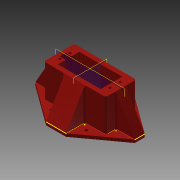
# Autodesk Inventor part: Servo Mount
Saved by Autodesk Inventor 2015 (Build 190159000, 159)
## iProperties
Created: 2016-12-13
Part Number: Servo Mount
Material: Generic
Document SubType Name: Modeling
Designer: Rudge-Top
Density: 1 g/cm^3
Appearance: Orange-Red
Author: Rudge-Top
Autodesk Inventor part; units mm, degrees
ref_plane "YZ Plane" through (0, 0, 0) normal (1, 0, 0) x (0, 1, 0)
ref_plane "XZ Plane" through (0, 0, 0) normal (0, 1, 0) x (-1, 0, 0)
ref_plane "XY Plane" through (0, 0, 0) normal (0, 0, 1) x (1, 0, 0)
sketch "Sketch1" plane through (0, 0, 0) normal (0, 1, 0) x (-1, 0, 0)
  line L0 (0, 0) -> (43, 0)
  line L1 (43, 0) -> (43, -21.5)
  line L2 (43, -21.5) -> (0, -21.5)
  line L3 (0, -21.5) -> (0, 0)
  line L4 (52.5, -26) -> (52.5, 4.5)
  line L5 (-9.5, 4.5) -> (-9.5, -26)
  line L6 (-9.5, 4.5) -> (52.5, 4.5)
  line L7 (52.5, -26) -> (-9.5, -26)
  dimension "d0" = 43
  dimension "d1" = 21.5
  dimension "d2" = 9.5
  dimension "d15" = 4.5
  dimension "d16" = 4.5
  dimension "d49" = 9.5
  constraints: 16 end point, 3 parallel, 3 perpendicular, 1 horizontal
  measures "d0" distance of L1.end L2.end
  measures "d1" distance of L0.end L1.end
  measures "d2" distance between parallel lines of L1 L4
  measures "d15" distance between parallel lines of L2 L7
  measures "d16" distance between parallel lines of L6 L0
  measures "d49" distance between parallel lines of L5 L3
extrude "Extrusion1" add sketch "Sketch1" along normal blind 29.5
sketch "Sketch2" plane through (0, 0, 0) normal (0, -1, 0) x (1, 0, 0)
  line L0 (-52.5, 4.5) -> (9.5, 4.5)
  line L1 (9.5, 4.5) -> (9.5, -26)
  line L2 (9.5, -26) -> (-52.5, -26)
  line L3 (-52.5, -26) -> (-52.5, 4.5)
  point P0 (0, 0)
  constraints: 8 end point, 2 parallel, 1 horizontal, 1 perpendicular
extrude "Extrusion2" add sketch "Sketch2" along normal blind 3
fillet "Fillet1" radius 2 4 edges at (-52.5, 13.25, -26) (9.5, 13.25, -26) (9.5, 13.25, 4.5) (-52.5, 13.25, 4.5)
sketch "Sketch3" plane through (0, 29.5, 0) normal (0, 1, 0) x (1, 0, 0)
  arc A0 (-52.5, -2.5) -> (-50.5, -4.5) centre (-50.5, -2.5) ccw projected
  arc A1 (7.5, -4.5) -> (9.5, -2.5) centre (7.5, -2.5) ccw projected
  line L0 (9.5, -2.5) -> (9.5, 24) projected
  arc A2 (9.5, 24) -> (7.5, 26) centre (7.5, 24) ccw projected
  arc A3 (-50.5, 26) -> (-52.5, 24) centre (-50.5, 24) ccw projected
  line L1 (-52.5, 24) -> (-52.5, -2.5) projected
  line L2 (-43, 0) -> (-43, 21.5) projected
  line L3 (-43, 21.5) -> (0, 21.5) projected
  line L4 (0, 21.5) -> (0, 0) projected
  line L5 (0, 0) -> (-43, 0) projected
  line L6 (-50.5, -4.5) -> (7.5, -4.5) projected
  line L7 (7.5, 26) -> (-50.5, 26) projected
  point P0 (3.5, 5.75)
  point P1 (3.5, 15.75)
  point P2 (-46.5, 5.75)
  point P3 (-46.5, 15.75)
  dimension "d8" = 10
  dimension "d10" = 3.5
  dimension "d11" = 10
  dimension "d12" = 3.5
  dimension "d17" = 10.25
  dimension "d18" = 10.25
  measures "d8" distance of point (-46.5, 5.75) point (-46.5, 15.75)
  measures "d10" distance from line of L2 point (-46.5, 15.75)
  measures "d11" distance of point (3.5, 15.75) point (3.5, 5.75)
  measures "d12" distance from line of L4 point (3.5, 5.75)
  measures "d17" distance from line of L6 point (3.5, 5.75)
  measures "d18" distance from line of L7 point (-46.5, 15.75)
hole "Hole1" at (3.5, 29.5, -5.75) at (3.5, 29.5, -15.75) at (-46.5, 29.5, -5.75) at (-46.5, 29.5, -15.75) direction (0, -1, 0) diameter 2.5 depth 20 tip angle 118
ref_plane "Work Plane1" through (-21.5, -3, 2.5) normal (1, 0, 0) x (0, 0, -1)
sketch "Sketch4" plane through (-21.5, -3, 2.5) normal (1, 0, 0) x (0, 0, -1)
  line L0 (0, 0) -> (0, 32.5) projected
  line L1 (26.5, 0) -> (0, 0) projected
  line L2 (26.5, 32.5) -> (26.5, 0) projected
  line L3 (0, 32.5) -> (26.5, 32.5) projected
  line L4 (28.5, 32.5) -> (26.5, 32.5) projected
  line L5 (26.5, 32.5) -> (26.5, 0) projected
  line L6 (26.5, 0) -> (28.5, 0) projected
  line L7 (28.5, 0) -> (28.5, 32.5) projected
  line L8 (28.5, 32.5) -> (47.2639, 0)
  line L9 (28.5, 32.5) -> (66.0278, 32.5) construction
  line L10 (47.2639, 0) -> (28.5, 0)
  point P0 (2.5, 3)
  dimension "d26" = 60
  constraints: 6 end point, 2 horizontal, 1 equal length
  measures "d26" angle of L8 L9
extrude "Extrusion3" add sketch "Sketch4" along normal mid plane 20 contours L7 L8 L10
ref_plane "Work Plane2" through (-50.5, -3, -10.75) normal (0, 0, -1) x (-1, 0, 0)
mirror "Mirror1" about plane through (-50.5, -3, -10.75) normal (0, 0, -1) of "Extrusion3"
sketch "Sketch5" plane through (-50.5, -3, -10.75) normal (0, 0, -1) x (-1, 0, 0)
  line L0 (-58, 32.5) -> (-60, 32.5) projected
  line L1 (-60, 32.5) -> (-60, 0) projected
  line L2 (-60, 0) -> (-58, 0) projected
  line L3 (-58, 0) -> (-58, 32.5) projected
  line L4 (-60, 32.5) -> (-78.7639, 0)
  line L5 (-60, 32.5) -> (-22.4722, 32.5) construction
  line L6 (-78.7639, 0) -> (-60, 0)
  line L7 (-60, 32.5) -> (-60, 0)
  point P0 (-50.5, 3)
  dimension "d29" = 240
  constraints: 8 end point, 2 horizontal, 1 collinear, 1 equal length
extrude "Extrusion4" add sketch "Sketch5" along normal mid plane 10 contours L1 L6 L4
mirror "Mirror2" about plane through (-21.5, -3, 2.5) normal (1, 0, 0) of "Extrusion4"
fillet "Fillet2" radius 2 8 edges at (9.5, 13.25, -15.75) (9.5, 13.25, -5.75) (-11.5, 13.25, -26) (-31.5, 13.25, -26) (-52.5, 13.25, -15.75) (-52.5, 13.25, -5.75) (-31.5, 13.25, 4.5) (-11.5, 13.25, 4.5)
sketch "Sketch6" plane through (0, -3, 0) normal (0, -1, 0) x (1, 0, 0)
  line L0 (-43, -21.5) -> (0, -21.5)
  line L1 (0, -21.5) -> (0, 0)
  line L2 (0, 0) -> (-43, 0)
  line L3 (-43, 0) -> (-43, -21.5)
  line L4 (-50.5, -26) -> (-33.5, -26) projected
  line L5 (-52.5, 2.5) -> (-52.5, -3.75) projected
  point P0 (0, 0)
  dimension "d33" = 43
  dimension "d34" = 21.5
  dimension "d35" = 4.5
  dimension "d36" = 9.5
  constraints: 8 end point, 2 parallel, 1 horizontal, 1 perpendicular
  measures "d33" distance of L2.end L1.end
  measures "d34" distance of L1.end L0.end
  measures "d35" distance between parallel lines of L4 L0
  measures "d36" distance between parallel lines of L5 L3
extrude "Extrusion5" cut sketch "Sketch6" against normal blind 3
sketch "Sketch7" plane through (0, 29.5, 0) normal (0, 1, 0) x (1, 0, 0)
  circle A0 centre (-46.5, 5.75) radius 1.25 projected
  circle A1 centre (3.5, 5.75) radius 1.25 projected
  circle A2 centre (3.5, 15.75) radius 1.25 projected
  circle A3 centre (-46.5, 15.75) radius 1.25 projected
  arc A4 (-52.5, -2.5) -> (-50.5, -4.5) centre (-50.5, -2.5) ccw projected
  line L0 (-50.5, -4.5) -> (-33.5, -4.5) projected
  line L1 (-33.5, -4.5) -> (-9.5, -4.5) projected
  line L2 (-9.5, -4.5) -> (7.5, -4.5) projected
  arc A5 (7.5, -4.5) -> (9.5, -2.5) centre (7.5, -2.5) ccw projected
  line L3 (9.5, -2.5) -> (9.5, 3.75) projected
  line L4 (9.5, 3.75) -> (9.5, 17.75) projected
  line L5 (9.5, 17.75) -> (9.5, 24) projected
  arc A6 (9.5, 24) -> (7.5, 26) centre (7.5, 24) ccw projected
  line L6 (7.5, 26) -> (-9.5, 26) projected
  line L7 (-9.5, 26) -> (-33.5, 26) projected
  line L8 (-33.5, 26) -> (-50.5, 26) projected
  arc A7 (-50.5, 26) -> (-52.5, 24) centre (-50.5, 24) ccw projected
  line L9 (-52.5, 24) -> (-52.5, 17.75) projected
  line L10 (-52.5, 17.75) -> (-52.5, 3.75) projected
  line L11 (-52.5, 3.75) -> (-52.5, -2.5) projected
  line L12 (-43, 0) -> (-43, 21.5) projected
  line L13 (-43, 21.5) -> (0, 21.5) projected
  line L14 (0, 21.5) -> (0, 0) projected
  line L15 (0, 0) -> (-43, 0) projected
  line L16 (-43, 13.75) -> (-49, 13.75)
  line L17 (-49, 13.75) -> (-49, 7.75)
  line L18 (-49, 7.75) -> (-43, 7.75)
  line L19 (-43, 7.75) -> (-43, 13.75)
  line L20 (-43, 10.75) -> (-46.1833, 10.75)
  line L21 (-43, 10.75) -> (-39.8167, 10.75) construction
  dimension "d39" = 6
  dimension "d40" = 6
  dimension "d41" = 180
  dimension "d51" = 7.75
  dimension "d52" = 7.75
  constraints: 12 end point, 2 horizontal, 2 parallel, 1 collinear, 1 midpoint, 1 perpendicular, 1 point on line
  measures "d39" distance of L18.end L17.end
  measures "d40" distance of L17.end L16.end
  measures "d41" angle of L20 L21
  measures "d51" distance from line of L13 L16.start
  measures "d52" distance from line of L15 L18.end
extrude "Extrusion6" cut sketch "Sketch7" against normal blind 40 contours L18 L17 L16 L12
fillet "Fillet3" radius 0.5 2 edges at (-43, 13.25, -13.75) (-43, 13.25, -7.75)
fillet "Fillet4" radius 0.5 4 edges at (0, 13.25, -21.5) (0, 13.25, 0) (-43, 13.25, -21.5) (-43, 13.25, 0)
sketch "Sketch8" plane through (0, -3, 0) normal (0, -1, 0) x (1, 0, 0)
  arc A0 (-50.5, 4.5) -> (-52.5, 2.5) centre (-50.5, 2.5) ccw projected
  line L0 (-52.5, 2.5) -> (-52.5, -3.75) projected
  arc A1 (-54.5, -5.75) -> (-52.5, -3.75) centre (-54.5, -3.75) ccw projected
  line L1 (-54.5, -5.75) -> (-71.2639, -5.75) projected
  line L2 (-71.2639, -5.75) -> (-71.2639, -15.75) projected
  line L3 (-71.2639, -15.75) -> (-54.5, -15.75) projected
  arc A2 (-52.5, -17.75) -> (-54.5, -15.75) centre (-54.5, -17.75) ccw projected
  line L4 (-52.5, -17.75) -> (-52.5, -24) projected
  arc A3 (-52.5, -24) -> (-50.5, -26) centre (-50.5, -24) ccw projected
  line L5 (-50.5, -26) -> (-33.5, -26) projected
  arc A4 (-31.5, -28) -> (-33.5, -26) centre (-33.5, -28) ccw projected
  line L6 (-31.5, -44.7639) -> (-31.5, -28) projected
  line L7 (-31.5, -44.7639) -> (-11.5, -44.7639) projected
  line L8 (-11.5, -28) -> (-11.5, -44.7639) projected
  arc A5 (-9.5, -26) -> (-11.5, -28) centre (-9.5, -28) ccw projected
  line L9 (-9.5, -26) -> (7.5, -26) projected
  arc A6 (7.5, -26) -> (9.5, -24) centre (7.5, -24) ccw projected
  line L10 (9.5, -24) -> (9.5, -17.75) projected
  arc A7 (11.5, -15.75) -> (9.5, -17.75) centre (11.5, -17.75) ccw projected
  line L11 (28.2639, -15.75) -> (11.5, -15.75) projected
  line L12 (28.2639, -5.75) -> (28.2639, -15.75) projected
  line L13 (11.5, -5.75) -> (28.2639, -5.75) projected
  arc A8 (9.5, -3.75) -> (11.5, -5.75) centre (11.5, -3.75) ccw projected
  line L14 (9.5, -3.75) -> (9.5, 2.5) projected
  arc A9 (9.5, 2.5) -> (7.5, 4.5) centre (7.5, 2.5) ccw projected
  line L15 (7.5, 4.5) -> (-9.5, 4.5) projected
  arc A10 (-11.5, 6.5) -> (-9.5, 4.5) centre (-9.5, 6.5) ccw projected
  line L16 (-11.5, 6.5) -> (-11.5, 23.2639) projected
  line L17 (-31.5, 23.2639) -> (-11.5, 23.2639) projected
  line L18 (-31.5, 23.2639) -> (-31.5, 6.5) projected
  arc A11 (-33.5, 4.5) -> (-31.5, 6.5) centre (-33.5, 6.5) ccw projected
  line L19 (-33.5, 4.5) -> (-50.5, 4.5) projected
  line L20 (-43, -7.25) -> (-43, -0.5) projected
  arc A12 (-42.5, 0) -> (-43, -0.5) centre (-42.5, -0.5) ccw projected
  line L21 (-42.5, 0) -> (-0.5, 0) projected
  arc A13 (0, -0.5) -> (-0.5, 0) centre (-0.5, -0.5) ccw projected
  line L22 (0, -0.5) -> (0, -21) projected
  arc A14 (-0.5, -21.5) -> (0, -21) centre (-0.5, -21) ccw projected
  line L23 (-0.5, -21.5) -> (-42.5, -21.5) projected
  arc A15 (-43, -21) -> (-42.5, -21.5) centre (-42.5, -21) ccw projected
  line L24 (-43.5, -13.75) -> (-49, -13.75) projected
  line L25 (-49, -13.75) -> (-49, -7.75) projected
  line L26 (-49, -7.75) -> (-43.5, -7.75) projected
  line L27 (-49, -13.75) -> (-71.2639, -13.75)
  line L28 (-71.2639, -13.75) -> (-71.2639, -7.75)
  line L29 (-71.2639, -7.75) -> (-49, -7.75)
  line L30 (-49, -7.75) -> (-49, -13.75)
  arc A16 (-43.5, -7.75) -> (-43, -7.25) centre (-43.5, -7.25) ccw projected
  line L31 (-43, -21) -> (-43, -14.25) projected
  arc A17 (-43, -14.25) -> (-43.5, -13.75) centre (-43.5, -14.25) ccw projected
  point P0 (0, 0)
  dimension "d50" = 6
  constraints: 8 end point, 2 parallel, 1 horizontal, 1 perpendicular, 1 point on line
  measures "d50" distance between parallel lines of L27 L29
extrude "Extrusion7" cut sketch "Sketch8" against normal blind 4 contours L29 L25 L27 L2
fillet "Fillet5" radius 2 2 edges at (-58.9772, 1, -13.75) (-58.9772, 1, -7.75)
sketch "Sketch9" plane through (0, -3, 0) normal (0, -1, 0) x (1, 0, 0)
  line L0 (-71.2639, -7.75) -> (-43.5, -7.75) projected
  arc A0 (-43.5, -7.75) -> (-43, -7.25) centre (-43.5, -7.25) ccw projected
  line L1 (-43, -7.25) -> (-43, -0.5) projected
  arc A1 (-42.5, 0) -> (-43, -0.5) centre (-42.5, -0.5) ccw projected
  line L2 (-42.5, 0) -> (-0.5, 0) projected
  arc A2 (0, -0.5) -> (-0.5, 0) centre (-0.5, -0.5) ccw projected
  line L3 (0, -0.5) -> (0, -21) projected
  arc A3 (-0.5, -21.5) -> (0, -21) centre (-0.5, -21) ccw projected
  line L4 (-0.5, -21.5) -> (-42.5, -21.5) projected
  arc A4 (-43, -21) -> (-42.5, -21.5) centre (-42.5, -21) ccw projected
  line L5 (-43, -21) -> (-43, -14.25) projected
  arc A5 (-43, -14.25) -> (-43.5, -13.75) centre (-43.5, -14.25) ccw projected
  line L6 (-43.5, -13.75) -> (-71.2639, -13.75) projected
  line L7 (-71.2639, -13.75) -> (-71.2639, -15.75) projected
  line L8 (-71.2639, -15.75) -> (-54.5, -15.75) projected
  arc A6 (-52.5, -17.75) -> (-54.5, -15.75) centre (-54.5, -17.75) ccw projected
  line L9 (-52.5, -17.75) -> (-52.5, -24) projected
  arc A7 (-52.5, -24) -> (-50.5, -26) centre (-50.5, -24) ccw projected
  line L10 (-50.5, -26) -> (-33.5, -26) projected
  arc A8 (-31.5, -28) -> (-33.5, -26) centre (-33.5, -28) ccw projected
  line L11 (-31.5, -44.7639) -> (-31.5, -28) projected
  line L12 (-31.5, -44.7639) -> (-11.5, -44.7639) projected
  line L13 (-11.5, -28) -> (-11.5, -44.7639) projected
  arc A9 (-9.5, -26) -> (-11.5, -28) centre (-9.5, -28) ccw projected
  line L14 (-9.5, -26) -> (7.5, -26) projected
  arc A10 (7.5, -26) -> (9.5, -24) centre (7.5, -24) ccw projected
  line L15 (9.5, -24) -> (9.5, -17.75) projected
  arc A11 (11.5, -15.75) -> (9.5, -17.75) centre (11.5, -17.75) ccw projected
  line L16 (28.2639, -15.75) -> (11.5, -15.75) projected
  line L17 (28.2639, -5.75) -> (28.2639, -15.75) projected
  line L18 (11.5, -5.75) -> (28.2639, -5.75) projected
  arc A12 (9.5, -3.75) -> (11.5, -5.75) centre (11.5, -3.75) ccw projected
  line L19 (9.5, -3.75) -> (9.5, 2.5) projected
  arc A13 (9.5, 2.5) -> (7.5, 4.5) centre (7.5, 2.5) ccw projected
  line L20 (7.5, 4.5) -> (-9.5, 4.5) projected
  arc A14 (-11.5, 6.5) -> (-9.5, 4.5) centre (-9.5, 6.5) ccw projected
  line L21 (-11.5, 6.5) -> (-11.5, 23.2639) projected
  line L22 (-31.5, 23.2639) -> (-11.5, 23.2639) projected
  line L23 (-31.5, 23.2639) -> (-31.5, 6.5) projected
  arc A15 (-33.5, 4.5) -> (-31.5, 6.5) centre (-33.5, 6.5) ccw projected
  line L24 (-33.5, 4.5) -> (-50.5, 4.5) projected
  arc A16 (-50.5, 4.5) -> (-52.5, 2.5) centre (-50.5, 2.5) ccw projected
  line L25 (-52.5, 2.5) -> (-52.5, -3.75) projected
  arc A17 (-54.5, -5.75) -> (-52.5, -3.75) centre (-54.5, -3.75) ccw projected
  line L26 (-54.5, -5.75) -> (-71.2639, -5.75) projected
  line L27 (-71.2639, -5.75) -> (-71.2639, -7.75) projected
  point P0 (0, 0)
sketch "Sketch10" plane through (0, -3, 0) normal (0, -1, 0) x (1, 0, 0)
  line L0 (-43.5, -13.75) -> (-71.2639, -13.75) projected
  line L1 (-71.2639, -13.75) -> (-71.2639, -15.75) projected
  line L2 (-71.2639, -15.75) -> (-54.5, -15.75) projected
  arc A0 (-52.5, -17.75) -> (-54.5, -15.75) centre (-54.5, -17.75) ccw projected
  line L3 (-52.5, -17.75) -> (-52.5, -24) projected
  arc A1 (-52.5, -24) -> (-50.5, -26) centre (-50.5, -24) ccw projected
  line L4 (-50.5, -26) -> (-33.5, -26) projected
  arc A2 (-31.5, -28) -> (-33.5, -26) centre (-33.5, -28) ccw projected
  line L5 (-31.5, -44.7639) -> (-31.5, -28) projected
  line L6 (-31.5, -44.7639) -> (-11.5, -44.7639) projected
  line L7 (-11.5, -28) -> (-11.5, -44.7639) projected
  arc A3 (-9.5, -26) -> (-11.5, -28) centre (-9.5, -28) ccw projected
  line L8 (-9.5, -26) -> (7.5, -26) projected
  arc A4 (7.5, -26) -> (9.5, -24) centre (7.5, -24) ccw projected
  line L9 (9.5, -24) -> (9.5, -17.75) projected
  arc A5 (11.5, -15.75) -> (9.5, -17.75) centre (11.5, -17.75) ccw projected
  line L10 (28.2639, -15.75) -> (11.5, -15.75) projected
  line L11 (28.2639, -5.75) -> (28.2639, -15.75) projected
  line L12 (11.5, -5.75) -> (28.2639, -5.75) projected
  arc A6 (9.5, -3.75) -> (11.5, -5.75) centre (11.5, -3.75) ccw projected
  line L13 (9.5, -3.75) -> (9.5, 2.5) projected
  arc A7 (9.5, 2.5) -> (7.5, 4.5) centre (7.5, 2.5) ccw projected
  line L14 (7.5, 4.5) -> (-9.5, 4.5) projected
  arc A8 (-11.5, 6.5) -> (-9.5, 4.5) centre (-9.5, 6.5) ccw projected
  line L15 (-11.5, 6.5) -> (-11.5, 23.2639) projected
  line L16 (-31.5, 23.2639) -> (-11.5, 23.2639) projected
  line L17 (-31.5, 23.2639) -> (-31.5, 6.5) projected
  arc A9 (-33.5, 4.5) -> (-31.5, 6.5) centre (-33.5, 6.5) ccw projected
  line L18 (-33.5, 4.5) -> (-50.5, 4.5) projected
  arc A10 (-50.5, 4.5) -> (-52.5, 2.5) centre (-50.5, 2.5) ccw projected
  line L19 (-52.5, 2.5) -> (-52.5, -3.75) projected
  arc A11 (-54.5, -5.75) -> (-52.5, -3.75) centre (-54.5, -3.75) ccw projected
  line L20 (-54.5, -5.75) -> (-71.2639, -5.75) projected
  line L21 (-71.2639, -5.75) -> (-71.2639, -7.75) projected
  line L22 (-71.2639, -7.75) -> (-43.5, -7.75) projected
  arc A12 (-43.5, -7.75) -> (-43, -7.25) centre (-43.5, -7.25) ccw projected
  line L23 (-43, -7.25) -> (-43, -0.5) projected
  arc A13 (-42.5, 0) -> (-43, -0.5) centre (-42.5, -0.5) ccw projected
  line L24 (-42.5, 0) -> (-0.5, 0) projected
  arc A14 (0, -0.5) -> (-0.5, 0) centre (-0.5, -0.5) ccw projected
  line L25 (0, -0.5) -> (0, -21) projected
  arc A15 (-0.5, -21.5) -> (0, -21) centre (-0.5, -21) ccw projected
  line L26 (-0.5, -21.5) -> (-42.5, -21.5) projected
  arc A16 (-43, -21) -> (-42.5, -21.5) centre (-42.5, -21) ccw projected
  line L27 (-43, -21) -> (-43, -14.25) projected
  arc A17 (-43, -14.25) -> (-43.5, -13.75) centre (-43.5, -14.25) ccw projected
  line L28 (-31.5, -44.7639) -> (-71.2639, -15.75)
  line L29 (28.2639, -15.75) -> (-11.5, -44.7639)
  line L30 (-71.2639, -5.75) -> (-31.5, 23.2639)
  line L31 (-11.5, 23.2639) -> (28.2639, -5.75)
  point P0 (0, 0)
  constraints: 8 end point, 1 parallel
extrude "Extrusion8" add sketch "Sketch10" along normal blind 3
fillet "Fillet7" radius 0.5 28 edges at (-10.9142, -3, 5.0858) (-1, -3, 4.5) (8.9142, -3, 3.9142) (9.5, -3, -0.625) (10.0858, -3, -5.1642) (19.8819, -3, -5.75) (-11.5, -3, 14.8819) (-1, -3, -26) (-10.9142, -3, -26.5858) (-11.5, -3, -36.3819) (9.5, -3, -20.875) (10.0858, -3, -16.3358) (19.8819, -3, -15.75) (8.9142, -3, -25.4142) (-32.0858, -3, -26.5858) (-31.5, -3, -36.3819) (-51.9142, -3, -25.4142) (-52.5, -3, -20.875) (-53.0858, -3, -16.3358) (-62.8819, -3, -15.75) (-42, -3, -26) (-53.0858, -3, -5.1642) (-52.5, -3, -0.625) (-51.9142, -3, 3.9142) (-42, -3, 4.5) (-32.0858, -3, 5.0858) (-31.5, -3, 14.8819) (-62.8819, -3, -5.75)
sketch "Sketch11" plane through (0, -3, 0) normal (0, 1, 0) x (1, 0, 0)
  line L0 (-11.5, 44.4752) -> (-11.5, 28) projected
  line L1 (7.5, 26) -> (-9.5, 26) projected
  line L2 (-11, 28) -> (-11, 44.3991) projected
  arc A0 (-11, 28) -> (-9.5, 26.5) centre (-9.5, 28) ccw projected
  line L3 (7.5, 26.5) -> (-9.5, 26.5) projected
  arc A1 (10, 24) -> (7.5, 26.5) centre (7.5, 24) ccw projected
  line L4 (10, 17.75) -> (10, 24) projected
  arc A2 (10, 17.75) -> (11.5, 16.25) centre (11.5, 17.75) ccw projected
  line L5 (27.5786, 16.25) -> (11.5, 16.25) projected
  line L6 (-11, 44.3991) -> (27.5786, 16.25) projected
  point P0 (0, 0)
  point P1 (-4, 31.8641)
  dimension "d57" = 7.5
  dimension "d59" = 6
  measures "d57" distance from line of point (-4, 31.864) L0
  measures "d59" distance from line of L6 point (-4, 31.864)
hole "Hole2" at (-4, -3, -31.8641) direction (0, -1, 0) diameter 3 end through all
mirror "Mirror3" about plane through (-21.5, -3, 2.5) normal (1, 0, 0) of "Hole2"
mirror "Mirror4" about plane through (-50.5, -3, -10.75) normal (0, 0, -1) of "Hole2", "Mirror3"
sketch "Sketch12" plane through (0, -3, 0) normal (0, 1, 0) x (1, 0, 0)
  line L0 (-64.6351, 20.7123) -> (-54.1295, 20.7123) construction
  line L1 (-54.1295, 20.7123) -> (-54.1295, 11.3759) construction
  line L2 (-54.1295, 11.3759) -> (-64.6351, 11.3759) construction
  line L3 (-64.6351, 11.3759) -> (-64.6351, 20.7123) construction
  line L4 (-62.1279, 18.3412) -> (-62.5448, 18.3412)
  line L5 (-62.5448, 18.3412) -> (-62.5448, 17.1386)
  line L6 (-62.5448, 17.1386) -> (-62.9958, 17.1386)
  line L7 (-62.9958, 17.1386) -> (-62.9958, 18.3412)
  line L8 (-62.9958, 18.3412) -> (-64.5415, 18.3412)
  line L9 (-64.5415, 18.3412) -> (-64.5415, 18.8347)
  line L10 (-64.5415, 18.8347) -> (-62.9759, 20.6386)
  line L11 (-62.9759, 20.6386) -> (-62.5448, 20.6386)
  line L12 (-62.5448, 20.6386) -> (-62.5448, 18.7184)
  line L13 (-62.5448, 18.7184) -> (-62.1279, 18.7184)
  line L14 (-62.1279, 18.7184) -> (-62.1279, 18.3412)
  line L15 (-62.9958, 18.7184) -> (-62.9958, 20.0855)
  line L16 (-62.9958, 20.0855) -> (-64.1728, 18.7184)
  line L17 (-64.1728, 18.7184) -> (-62.9958, 18.7184)
  line L18 (-59.595, 17.1386) -> (-61.7535, 17.1386)
  line L19 (-61.7535, 17.1386) -> (-61.7535, 17.6349)
  spline S0 degree 2 poles (-61.7535, 17.6349) (-61.5209, 17.8533) (-61.1068, 18.2589) (-60.9082, 18.4773) knots 0 0 0 1 2 2 2
  spline S1 degree 2 poles (-60.9082, 18.4773) (-60.5083, 18.9169) (-60.2162, 19.4445) (-60.2162, 19.7253) knots 0 0 0 1 2 2 2
  spline S2 degree 2 poles (-60.2162, 19.7253) (-60.2162, 19.8728) (-60.3069, 20.094) (-60.3892, 20.1649) knots 0 0 0 1 2 2 2
  spline S3 degree 2 poles (-60.3892, 20.1649) (-60.4715, 20.2358) (-60.687, 20.3067) (-60.8175, 20.3067) knots 0 0 0 1 2 2 2
  spline S4 degree 2 poles (-60.8175, 20.3067) (-60.9423, 20.3067) (-61.1975, 20.2443) (-61.3138, 20.1961) knots 0 0 0 1 2 2 2
  spline S5 degree 2 poles (-61.3138, 20.1961) (-61.4131, 20.1564) (-61.5975, 20.0429) (-61.6542, 20.0032) knots 0 0 0 1 2 2 2
  line L20 (-61.6542, 20.0032) -> (-61.6797, 20.0032)
  line L21 (-61.6797, 20.0032) -> (-61.6797, 20.5024)
  spline S6 degree 2 poles (-61.6797, 20.5024) (-61.5351, 20.5733) (-61.016, 20.7123) (-60.7834, 20.7123) knots 0 0 0 1 2 2 2
  spline S7 degree 2 poles (-60.7834, 20.7123) (-60.2928, 20.7123) (-59.7397, 20.1933) (-59.7397, 19.7508) knots 0 0 0 1 2 2 2
  spline S8 degree 2 poles (-59.7397, 19.7508) (-59.7397, 19.5438) (-59.8361, 19.1977) (-59.9212, 19.0502) knots 0 0 0 1 2 2 2
  spline S9 degree 2 poles (-59.9212, 19.0502) (-60.0063, 18.8971) (-60.2531, 18.5964) (-60.3892, 18.4518) knots 0 0 0 1 2 2 2
  spline S10 degree 2 poles (-60.3892, 18.4518) (-60.6104, 18.2107) (-61.1522, 17.6945) (-61.3138, 17.5442) knots 0 0 0 1 2 2 2
  line L22 (-61.3138, 17.5442) -> (-59.595, 17.5442)
  line L23 (-59.595, 17.5442) -> (-59.595, 17.1386)
  spline S11 degree 2 poles (-56.9488, 18.8886) (-56.9488, 17.9469) (-57.4962, 17.0648) (-58.0663, 17.0648) knots 0 0 0 1 2 2 2
  spline S12 degree 2 poles (-58.0663, 17.0648) (-58.6449, 17.0648) (-59.1866, 17.9639) (-59.1866, 18.8857) knots 0 0 0 1 2 2 2
  spline S13 degree 2 poles (-59.1866, 18.8857) (-59.1866, 19.8331) (-58.6392, 20.7095) (-58.0663, 20.7095) knots 0 0 0 1 2 2 2
  spline S14 degree 2 poles (-58.0663, 20.7095) (-57.4905, 20.7095) (-56.9488, 19.8019) (-56.9488, 18.8886) knots 0 0 0 1 2 2 2
  spline S15 degree 2 poles (-57.5501, 17.8221) (-57.482, 17.9951) (-57.4253, 18.5284) (-57.4253, 18.8886) knots 0 0 0 1 2 2 2
  spline S16 degree 2 poles (-57.4253, 18.8886) (-57.4253, 19.2488) (-57.482, 19.7792) (-57.5529, 19.9579) knots 0 0 0 1 2 2 2
  spline S17 degree 2 poles (-57.5529, 19.9579) (-57.6238, 20.1365) (-57.8706, 20.3209) (-58.0663, 20.3209) knots 0 0 0 1 2 2 2
  spline S18 degree 2 poles (-58.0663, 20.3209) (-58.262, 20.3209) (-58.5144, 20.1365) (-58.5881, 19.9522) knots 0 0 0 1 2 2 2
  spline S19 degree 2 poles (-58.5881, 19.9522) (-58.6591, 19.7735) (-58.7101, 19.2289) (-58.7101, 18.8857) knots 0 0 0 1 2 2 2
  spline S20 degree 2 poles (-58.7101, 18.8857) (-58.7101, 18.517) (-58.6647, 18.0235) (-58.591, 17.8306) knots 0 0 0 1 2 2 2
  spline S21 degree 2 poles (-58.591, 17.8306) (-58.5229, 17.6491) (-58.2705, 17.4534) (-58.0663, 17.4534) knots 0 0 0 1 2 2 2
  spline S22 degree 2 poles (-58.0663, 17.4534) (-57.8734, 17.4534) (-57.621, 17.6378) (-57.5501, 17.8221) knots 0 0 0 1 2 2 2
  line L24 (-54.3422, 17.1386) -> (-56.5006, 17.1386)
  line L25 (-56.5006, 17.1386) -> (-56.5006, 17.6349)
  spline S23 degree 2 poles (-56.5006, 17.6349) (-56.268, 17.8533) (-55.8539, 18.2589) (-55.6554, 18.4773) knots 0 0 0 1 2 2 2
  spline S24 degree 2 poles (-55.6554, 18.4773) (-55.2555, 18.9169) (-54.9633, 19.4445) (-54.9633, 19.7253) knots 0 0 0 1 2 2 2
  spline S25 degree 2 poles (-54.9633, 19.7253) (-54.9633, 19.8728) (-55.0541, 20.094) (-55.1364, 20.1649) knots 0 0 0 1 2 2 2
  spline S26 degree 2 poles (-55.1364, 20.1649) (-55.2186, 20.2358) (-55.4342, 20.3067) (-55.5646, 20.3067) knots 0 0 0 1 2 2 2
  spline S27 degree 2 poles (-55.5646, 20.3067) (-55.6894, 20.3067) (-55.9447, 20.2443) (-56.061, 20.1961) knots 0 0 0 1 2 2 2
  spline S28 degree 2 poles (-56.061, 20.1961) (-56.1603, 20.1564) (-56.3446, 20.0429) (-56.4014, 20.0032) knots 0 0 0 1 2 2 2
  line L26 (-56.4014, 20.0032) -> (-56.4269, 20.0032)
  line L27 (-56.4269, 20.0032) -> (-56.4269, 20.5024)
  spline S29 degree 2 poles (-56.4269, 20.5024) (-56.2822, 20.5733) (-55.7632, 20.7123) (-55.5306, 20.7123) knots 0 0 0 1 2 2 2
  spline S30 degree 2 poles (-55.5306, 20.7123) (-55.0399, 20.7123) (-54.4868, 20.1933) (-54.4868, 19.7508) knots 0 0 0 1 2 2 2
  spline S31 degree 2 poles (-54.4868, 19.7508) (-54.4868, 19.5438) (-54.5833, 19.1977) (-54.6684, 19.0502) knots 0 0 0 1 2 2 2
  spline S32 degree 2 poles (-54.6684, 19.0502) (-54.7535, 18.8971) (-55.0002, 18.5964) (-55.1364, 18.4518) knots 0 0 0 1 2 2 2
  spline S33 degree 2 poles (-55.1364, 18.4518) (-55.3576, 18.2107) (-55.8993, 17.6945) (-56.061, 17.5442) knots 0 0 0 1 2 2 2
  line L28 (-56.061, 17.5442) -> (-54.3422, 17.5442)
  line L29 (-54.3422, 17.5442) -> (-54.3422, 17.1386)
  point P0 (0, 0)
  constraints: 2 other
extrude "Extrusion9" add sketch "Sketch12" along normal blind 1
ref_plane "Work Plane3" through (-21.5, -3, 2.5) normal (1, 0, 0) x (0, 0, -1)
body "Solid1"
